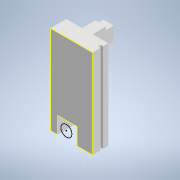
# Autodesk Inventor part: center_tray_top
Saved by Autodesk Inventor 2020 (Build 240168000, 168)
## iProperties
Created: 2022-09-22
Part Number: center_tray_top
Material: 일반
Document SubType Name: Modeling
Designer: SeungJin
Density: 1 g/cm^3
Appearance: 기본값
Author: SeungJin
Autodesk Inventor part; units mm, degrees
ref_plane "YZ Plane" through (0, 0, 0) normal (1, 0, 0) x (0, 1, 0)
ref_plane "XZ Plane" through (0, 0, 0) normal (0, 1, 0) x (-1, 0, 0)
ref_plane "XY Plane" through (0, 0, 0) normal (0, 0, 1) x (1, 0, 0)
sketch "스케치1" plane through (0, 0, 0) normal (0, 0, 1) x (1, 0, 0)
  line L0 (-62, -188.5) -> (-62, 261.5) projected
  line L1 (-32, -188.5) -> (-32, 261.5) projected
  line L2 (-12, -188.5) -> (-12, 261.5) projected
  line L3 (18, -188.5) -> (18, 261.5) projected
  line L4 (-292, 198.5399) -> (248, 198.5399) projected
  line L5 (-12, 192.5) -> (-32, 192.5) projected
  line L6 (-292, 30) -> (248, 30) projected
  line L7 (-292, 0) -> (248, 0) projected
  line L8 (-32, 167.5) -> (-11, 167.5)
  point P0 (0, 0)
  point P1 (-62, 30)
  point P2 (18, 30)
  point P3 (18, 198.5399)
  point P4 (-62, 198.5399)
  point P5 (-32, 30)
  point P6 (-12, 30)
  point P7 (-12, 167.5)
  dimension "d4" = 137.5
  constraints: 2 end point, 1 perpendicular, 1 point on line
  measures "d4" distance between parallel lines of L8 L6
extrude "돌출1" add sketch "스케치1" against normal blind 20 contours L1 L8 L2 L6
sketch "스케치2" plane through (0, 0, 0) normal (0, 0, 1) x (1, 0, 0)
  line L0 (-12, 192.5) -> (-32, 192.5) projected
  line L1 (-292, 198.5399) -> (248, 198.5399) projected
  line L2 (-32, -188.5) -> (-32, 261.5) projected
  line L3 (-12, -188.5) -> (-12, 261.5) projected
  point P0 (0, 0)
  point P1 (-12, 198.5399)
  point P2 (-32, 198.5399)
extrude "돌출2" add sketch "스케치2" against normal blind 25.3
sketch "스케치3" plane through (0, 0, 0) normal (0, 0, 1) x (1, 0, 0)
  line L0 (-12, 167.5) -> (-32, 167.5) projected
  line L1 (-32, -188.5) -> (-32, 261.5) projected
  line L2 (-32, 192.5) -> (-12, 192.5) projected
  line L3 (-12, -188.5) -> (-12, 261.5) projected
  point P0 (0, 0)
extrude "돌출3" add sketch "스케치3" against normal blind 40
sketch "스케치4" plane through (0, 0, 0) normal (0, 0, 1) x (1, 0, 0)
  line L0 (-62, -188.5) -> (-62, 261.5) projected
  line L1 (18, -188.5) -> (18, 261.5) projected
  line L2 (-292, 30) -> (248, 30) projected
  line L3 (-292, 198.5399) -> (248, 198.5399) projected
  point P0 (0, 0)
  point P1 (18, 198.5399)
  point P2 (-62, 198.5399)
  point P3 (-62, 30)
  point P4 (18, 30)
extrude "돌출4" add sketch "스케치4" along normal blind 30
sketch "스케치6" plane through (18, 30, 0) normal (1, 0, 0) x (0, 0, -1)
  line L0 (0, 0) -> (0, 168.5399) projected
  line L1 (0, 168.5399) -> (-30, 168.5399) projected
  line L2 (-30, 0) -> (-30, 168.5399) projected
  line L3 (0, 0) -> (-30, 0) projected
  line L4 (0, 0) -> (-30, 0) projected
  line L5 (-10, 0) -> (-10, 168.5399)
  line L6 (-15, 0) -> (-15, 168.5399)
  line L7 (0, 168.5399) -> (-30, 168.5399) projected
  point P0 (0, -30)
  point P1 (-15, 0)
  dimension "d9" = 10
  dimension "d10" = 15
  constraints: 4 end point, 2 midpoint, 2 perpendicular, 2 point on line
  measures "d9" distance between parallel lines of L5 L0
  measures "d10" distance between parallel lines of L0 L6
extrude "돌출5" cut sketch "스케치6" against normal blind 5 contours L3 L6 L1 L5
sketch "스케치7" plane through (0, 0, 30) normal (0, 0, 1) x (1, 0, 0)
  line L0 (-62, 198.5399) -> (-62, 30) projected
  line L1 (-62, 30) -> (18, 30) projected
  line L2 (18, 30) -> (18, 198.5399) projected
  line L3 (18, 198.5399) -> (-62, 198.5399) projected
  line L4 (-12, 167.5) -> (-12, 30) projected
  line L5 (-12, 30) -> (-32, 30) projected
  line L6 (-32, 30) -> (-32, 167.5) projected
  line L7 (-32, 167.5) -> (-12, 167.5) projected
  line L8 (-62, 62) -> (18, 62)
  line L9 (18, 30) -> (18, 198.5399) projected
  point P0 (0, 0)
  point P1 (-12, 62)
  point P2 (-32, 62)
  dimension "d13" = 32
  constraints: 2 end point, 2 point on line, 1 perpendicular
  measures "d13" distance between parallel lines of L1 L8
extrude "돌출6" cut sketch "스케치7" against normal through all contours L8 L4 L1 L6
sketch "스케치8" plane through (0, 0, 30) normal (0, 0, 1) x (1, 0, 0)
  line L0 (-32, 30) -> (-32, 62) projected
  line L1 (-32, 62) -> (-12, 62) projected
  line L2 (-12, 62) -> (-12, 30) projected
  line L3 (-12, 30) -> (18, 30) projected
  line L4 (18, 30) -> (18, 198.5399) projected
  line L5 (18, 198.5399) -> (-62, 198.5399) projected
  line L6 (-62, 198.5399) -> (-62, 30) projected
  line L7 (-62, 30) -> (-32, 30) projected
  line L8 (-32, 62) -> (-49, 62)
  line L9 (-49, 62) -> (-49, 30)
  line L10 (-49, 30) -> (-32, 30)
  line L11 (-32, 30) -> (-32, 62)
  point P0 (0, 0)
  dimension "d16" = 17
  constraints: 8 end point, 2 parallel, 1 horizontal, 1 perpendicular, 1 point on line
  measures "d16" distance of L10.end L9.end
extrude "돌출7" cut sketch "스케치8" against normal blind 30 contours L7 L9 L8 L0
sketch "스케치9" plane through (0, 0, 30) normal (0, 0, 1) x (1, 0, 0)
  line L0 (-49, 30) -> (-49, 62) projected
  line L1 (-49, 62) -> (-12, 62) projected
  line L2 (-12, 62) -> (-12, 30) projected
  line L3 (-12, 30) -> (18, 30) projected
  line L4 (18, 30) -> (18, 198.5399) projected
  line L5 (18, 198.5399) -> (-62, 198.5399) projected
  line L6 (-62, 198.5399) -> (-62, 30) projected
  line L7 (-62, 30) -> (-49, 30) projected
  circle A0 centre (-32.1, 44.85) radius 10.4999
  circle A1 centre (-32.1, 44.85) radius 10.4999
  circle A2 centre (-32.1, 44.85) radius 11
  line L8 (-49, 30) -> (-12, 30)
  point P0 (0, 0)
  dimension "d19" = 22
  constraints: 3 centre point, 2 end point, 1 coincident, 1 horizontal, 4 other
  measures "d19" diameter of A2
extrude "돌출8" add sketch "스케치9" against normal blind 12 contours L0 L1 L2 L8
sketch "스케치10" plane through (0, 0, 30) normal (0, 0, 1) x (1, 0, 0)
  circle A0 centre (-32.1, 44.85) radius 11 projected
  line L0 (-62, 30) -> (18, 30) projected
  line L1 (18, 30) -> (18, 198.5399) projected
  line L2 (18, 198.5399) -> (-62, 198.5399) projected
  line L3 (-62, 198.5399) -> (-62, 30) projected
  line L4 (-17.1, 44.85) -> (-17.1, 30)
  line L5 (-62, 30) -> (18, 30) projected
  line L6 (-47.1, 44.85) -> (-47.1, 29.85)
  arc A1 (-17.1, 44.85) -> (-47.1, 44.85) centre (-32.1, 44.85) ccw
  point P0 (0, 0)
  point P1 (-47.1, 30)
  constraints: 4 end point, 2 point on circle, 2 vertical, 1 centre point, 1 coincident, 1 point on line
extrude "돌출9" cut sketch "스케치10" against normal blind 2 contours L0 L6 A1 L4
